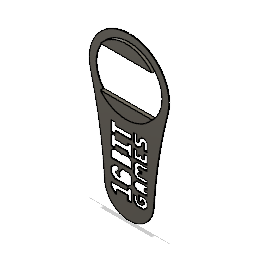
Poco X3 Phone Case Charm v1 (Autodesk Fusion 360 design; units mm, degrees)
Autodesk Fusion 360 part; units mm, degrees
note: some values were not read from the file. Chosen so that the rebuilt part matches the saved one: which pieces of a blend or face edit are solid. Set by a fixed rule: which sketch regions a step uses.
sketch "Sketch1" plane through (0, 0, 0) normal (0, 0, 1) x (1, 0, 0)
  circle A0 centre (0, 0) radius 18.4
  line L0 (-18.4, 0) -> (-13.8, 0)
  line L1 (-13.8, 0) -> (-13.8, -12.1705)
  line L2 (18.4, 0) -> (13.8, 0)
  line L3 (13.8, 0) -> (13.8, -12.1705)
  line L4 (0, -18.4) -> (0, -68.4)
  circle A1 centre (0, -54.6) radius 13.8
  line L5 (-13.8, -12.1705) -> (-13.8, -54.6)
  line L6 (13.8, -12.1705) -> (13.8, -54.6)
  circle A2 centre (0, 0) radius 22.4
  line L7 (-18.4, 0) -> (-22.4, 0)
  line L8 (18.4, 0) -> (22.4, 0)
  line L9 (0, 0) -> (0, 11.25)
  circle A3 centre (0, 0) radius 17.4
  line L10 (0, 11.25) -> (13.2739, 11.25)
  line L11 (13.2739, 11.25) -> (-13.2739, 11.25)
  line L12 (-13.2739, 11.25) -> (-13.2739, -11.25)
  line L13 (-13.2739, -11.25) -> (13.2739, -11.25)
  line L14 (13.2739, -11.25) -> (13.2739, 11.25)
  line L15 (-13.2739, 0) -> (-13.2739, -11.25)
  line L16 (-13.2739, -5.625) -> (-21.6822, -5.625)
  line L17 (-13.2739, -5.625) -> (21.6822, -5.625)
  arc A4 (-13.8, -54.6) -> (-21.6822, -5.625) centre (-276.7651, -71.8009) ccw
  arc A5 (21.6822, -5.625) -> (13.8, -54.6) centre (276.765, -71.8009) ccw
  dimension "d1" = 36.8
  dimension "d2" = 4.6
  dimension "d3" = 4.6
  dimension "d4" = 50
  dimension "d5" = 27.6
  dimension "d6" = 4
  dimension "d7" = 11.25
  dimension "d8" = -1
  dimension "d9" = 22.5
  constraint coincident A0.centre A2.centre
  constraint coincident A0 L0.start
  constraint horizontal L0
  constraint coincident A0 L1.end
  constraint perpendicular L0 L1
  constraint coincident A0 L2.start
  constraint perpendicular L1 L2
  constraint coincident A0 L3.end
  constraint perpendicular L2 L3
  constraint coincident A0 L4.start
  constraint vertical L4
  constraint coincident L4.end A1
  constraint coincident A1 L5.end
  constraint tangent A1 L5
  constraint parallel L1 L5
  constraint coincident A1 L6.end
  constraint tangent A1 L6
  constraint parallel L3 L6
  constraint coincident A2 L7.end
  constraint parallel L0 L7
  constraint coincident A2 L8.end
  constraint parallel L2 L8
  constraint vertical L9
  constraint coincident A3 L10.end
  constraint perpendicular L9 L10
  constraint horizontal L11
  constraint vertical L12
  constraint horizontal L13
  constraint vertical L14
  constraint coincident A3 L12.end
  constraint midpoint L12 L15.start
  constraint midpoint L15 L16.start
  constraint coincident A2 L16.end
  constraint perpendicular L15 L16
  constraint coincident A2 L17.end
  constraint parallel L16 L17
  constraint tangent A2 A4
  constraint tangent A2 A5
  measures "d1" diameter of A0
  measures "d2" distance of L0.start L0.end
  measures "d3" distance of L2.start L2.end
  measures "d4" distance of L4.start L4.end
  measures "d5" diameter of A1
  measures "d7" distance of A0.centre L9.end
  measures "d9" distance of L10.end L13.end
extrude "Extrude1" add sketch "Sketch1" along normal blind 0.8 contours A0 L0 L2 A3 | A0 A2 L8 L17 | A0 L2 A3 L17 | A0 A2 L7 L8 | A0 L0 A3 L16 | A0 A2 L7 L16 | A0 L6 A2 L17 | A0 L3 A3 L17 | A0 L1 A3 L16 | A0 L5 A2 L16 | A0 L4 L6 A2 | A0 L1 L3 A3 | L6 A2 A5 | A3 L10 L11 | A0 L4 L5 A2 | L5 A2 A4 | L4 A1 L6 A2 | L4 A1 | L4 A1 L5 A2 | L4 A1 | A3 L13 makes body 1
extrude "Extrude2" add sketch "Sketch1" along normal blind 2 contours A0 L0 L2 A3 | A0 L2 A3 L17 | A0 L0 A3 L16 | A0 L3 A3 L17 | A0 L1 A3 L16 | A0 L1 L3 A3 | A3 L10 L11 | A3 L13 bodies 1
extrude "Extrude3" cut 1 faces at (-0.4583, -31.5299, 0.8) along direction (0, 0, -1) blind 0.4 on bodies 1 bodies 1
sketch "Sketch2" plane through (0, 0, 0.4) normal (0, 0, 1) x (1, 0, 0)
  circle A0 centre (0, 0) radius 18.4
  arc A1 (-13.8, -54.6) -> (13.8, -54.6) centre (0, -54.6) ccw
  arc A2 (21.6822, -5.625) -> (13.8, -54.6) centre (276.765, -71.8009) ccw
  arc A3 (21.6822, -5.625) -> (-21.6822, -5.625) centre (0, 0) ccw
  arc A4 (-13.8, -54.6) -> (-21.6822, -5.625) centre (-276.7651, -71.8009) ccw
  line L0 (-10.0235, -64.9162) -> (-9.6068, -64.9162)
  line L1 (-9.6068, -64.9162) -> (-9.6068, -65.3329)
  line L2 (-9.6068, -65.3329) -> (-9.1902, -65.3329)
  line L3 (-9.1902, -65.3329) -> (-9.1902, -65.7495)
  line L4 (-9.1902, -65.7495) -> (-8.7735, -65.7495)
  line L5 (-8.7735, -65.7495) -> (-8.7735, -66.1662)
  line L6 (-8.7735, -66.1662) -> (-8.3568, -66.1662)
  line L7 (-8.3568, -66.1662) -> (-8.3568, -66.5829)
  line L8 (-8.3568, -66.5829) -> (-7.9402, -66.5829)
  line L9 (-7.9402, -66.5829) -> (-7.9402, -66.9995)
  line L10 (-7.9402, -66.9995) -> (-7.1068, -66.9995)
  line L11 (-7.1068, -66.9995) -> (-7.1068, -64.4995)
  line L12 (-7.1068, -64.4995) -> (-0.8568, -64.4995)
  line L13 (-0.8568, -64.4995) -> (-0.8568, -66.9995)
  line L14 (-0.8568, -66.9995) -> (1.2265, -66.9995)
  line L15 (1.2265, -66.9995) -> (1.2265, -60.7495)
  line L16 (1.2265, -60.7495) -> (-0.8568, -60.7495)
  line L17 (-0.8568, -60.7495) -> (-0.8568, -62.4162)
  line L18 (-0.8568, -62.4162) -> (-10.0235, -62.4162)
  line L19 (-10.0235, -62.4162) -> (-10.0235, -64.9162)
  line L20 (-10.0235, -58.2495) -> (-9.6068, -58.2495)
  line L21 (-9.6068, -58.2495) -> (-9.6068, -58.6662)
  line L22 (-9.6068, -58.6662) -> (-9.1902, -58.6662)
  line L23 (-9.1902, -58.6662) -> (-9.1902, -59.0829)
  line L24 (-9.1902, -59.0829) -> (-8.7735, -59.0829)
  line L25 (-8.7735, -59.0829) -> (-8.7735, -59.4995)
  line L26 (-8.7735, -59.4995) -> (-8.3568, -59.4995)
  line L27 (-8.3568, -59.4995) -> (-8.3568, -59.9162)
  line L28 (-8.3568, -59.9162) -> (-0.4402, -59.9162)
  line L29 (-0.4402, -59.9162) -> (-0.4402, -59.4995)
  line L30 (-0.4402, -59.4995) -> (-0.0235, -59.4995)
  line L31 (-0.0235, -59.4995) -> (-0.0235, -59.0829)
  line L32 (-0.0235, -59.0829) -> (0.3932, -59.0829)
  line L33 (0.3932, -59.0829) -> (0.3932, -58.6662)
  line L34 (0.3932, -58.6662) -> (0.8098, -58.6662)
  line L35 (0.8098, -58.6662) -> (0.8098, -58.2495)
  line L36 (0.8098, -58.2495) -> (1.2265, -58.2495)
  line L37 (1.2265, -58.2495) -> (1.2265, -54.4995)
  line L38 (1.2265, -54.4995) -> (0.8098, -54.4995)
  line L39 (0.8098, -54.4995) -> (0.8098, -54.0829)
  line L40 (0.8098, -54.0829) -> (0.3932, -54.0829)
  line L41 (0.3932, -54.0829) -> (0.3932, -53.6662)
  line L42 (0.3932, -53.6662) -> (-0.0235, -53.6662)
  line L43 (-0.0235, -53.6662) -> (-0.0235, -53.2495)
  line L44 (-0.0235, -53.2495) -> (-3.7735, -53.2495)
  line L45 (-3.7735, -53.2495) -> (-3.7735, -53.6662)
  line L46 (-3.7735, -53.6662) -> (-4.1902, -53.6662)
  line L47 (-4.1902, -53.6662) -> (-4.1902, -54.0829)
  line L48 (-4.1902, -54.0829) -> (-4.6068, -54.0829)
  line L49 (-4.6068, -54.0829) -> (-4.6068, -54.4995)
  line L50 (-4.6068, -54.4995) -> (-5.0235, -54.4995)
  line L51 (-5.0235, -54.4995) -> (-5.0235, -54.9162)
  line L52 (-5.0235, -54.9162) -> (-5.4402, -54.9162)
  line L53 (-5.4402, -54.9162) -> (-5.4402, -57.4162)
  line L54 (-5.4402, -57.4162) -> (-5.0235, -57.4162)
  line L55 (-5.0235, -57.4162) -> (-5.0235, -57.8329)
  line L56 (-5.0235, -57.8329) -> (-6.6902, -57.8329)
  line L57 (-6.6902, -57.8329) -> (-6.6902, -57.4162)
  line L58 (-6.6902, -57.4162) -> (-7.1068, -57.4162)
  line L59 (-7.1068, -57.4162) -> (-7.1068, -56.9995)
  line L60 (-7.1068, -56.9995) -> (-7.5235, -56.9995)
  line L61 (-7.5235, -56.9995) -> (-7.5235, -55.7495)
  line L62 (-7.5235, -55.7495) -> (-7.1068, -55.7495)
  line L63 (-7.1068, -55.7495) -> (-7.1068, -55.3329)
  line L64 (-7.1068, -55.3329) -> (-6.2735, -55.3329)
  line L65 (-6.2735, -55.3329) -> (-6.2735, -53.2495)
  line L66 (-6.2735, -53.2495) -> (-8.3568, -53.2495)
  line L67 (-8.3568, -53.2495) -> (-8.3568, -53.6662)
  line L68 (-8.3568, -53.6662) -> (-8.7735, -53.6662)
  line L69 (-8.7735, -53.6662) -> (-8.7735, -54.0829)
  line L70 (-8.7735, -54.0829) -> (-9.1902, -54.0829)
  line L71 (-9.1902, -54.0829) -> (-9.1902, -54.4995)
  line L72 (-9.1902, -54.4995) -> (-9.6068, -54.4995)
  line L73 (-9.6068, -54.4995) -> (-9.6068, -54.9162)
  line L74 (-9.6068, -54.9162) -> (-10.0235, -54.9162)
  line L75 (-10.0235, -54.9162) -> (-10.0235, -58.2495)
  line L76 (-10.0235, -50.7495) -> (1.2265, -50.7495)
  line L77 (1.2265, -50.7495) -> (1.2265, -46.9995)
  line L78 (1.2265, -46.9995) -> (0.8098, -46.9995)
  line L79 (0.8098, -46.9995) -> (0.8098, -46.5829)
  line L80 (0.8098, -46.5829) -> (0.3932, -46.5829)
  line L81 (0.3932, -46.5829) -> (0.3932, -46.1662)
  line L82 (0.3932, -46.1662) -> (-0.0235, -46.1662)
  line L83 (-0.0235, -46.1662) -> (-0.0235, -45.7495)
  line L84 (-0.0235, -45.7495) -> (-3.7735, -45.7495)
  line L85 (-3.7735, -45.7495) -> (-3.7735, -46.1662)
  line L86 (-3.7735, -46.1662) -> (-4.1902, -46.1662)
  line L87 (-4.1902, -46.1662) -> (-4.1902, -46.5829)
  line L88 (-4.1902, -46.5829) -> (-4.6068, -46.5829)
  line L89 (-4.6068, -46.5829) -> (-4.6068, -46.1662)
  line L90 (-4.6068, -46.1662) -> (-5.0235, -46.1662)
  line L91 (-5.0235, -46.1662) -> (-5.0235, -45.7495)
  line L92 (-5.0235, -45.7495) -> (-8.7735, -45.7495)
  line L93 (-8.7735, -45.7495) -> (-8.7735, -46.1662)
  line L94 (-8.7735, -46.1662) -> (-9.1902, -46.1662)
  line L95 (-9.1902, -46.1662) -> (-9.1902, -46.5829)
  line L96 (-9.1902, -46.5829) -> (-9.6068, -46.5829)
  line L97 (-9.6068, -46.5829) -> (-9.6068, -46.9995)
  line L98 (-9.6068, -46.9995) -> (-10.0235, -46.9995)
  line L99 (-10.0235, -46.9995) -> (-10.0235, -50.7495)
  line L100 (-10.0235, -44.9162) -> (-7.9402, -44.9162)
  line L101 (-7.9402, -44.9162) -> (-7.9402, -43.2495)
  line L102 (-7.9402, -43.2495) -> (-0.8568, -43.2495)
  line L103 (-0.8568, -43.2495) -> (-0.8568, -44.9162)
  line L104 (-0.8568, -44.9162) -> (1.2265, -44.9162)
  line L105 (1.2265, -44.9162) -> (1.2265, -39.0829)
  line L106 (1.2265, -39.0829) -> (-0.8568, -39.0829)
  line L107 (-0.8568, -39.0829) -> (-0.8568, -40.7495)
  line L108 (-0.8568, -40.7495) -> (-7.9402, -40.7495)
  line L109 (-7.9402, -40.7495) -> (-7.9402, -39.0829)
  line L110 (-7.9402, -39.0829) -> (-10.0235, -39.0829)
  line L111 (-10.0235, -39.0829) -> (-10.0235, -44.9162)
  line L112 (-10.0235, -38.2495) -> (-7.9402, -38.2495)
  line L113 (-7.9402, -38.2495) -> (-7.9402, -36.5829)
  line L114 (-7.9402, -36.5829) -> (1.2265, -36.5829)
  line L115 (1.2265, -36.5829) -> (1.2265, -34.0829)
  line L116 (1.2265, -34.0829) -> (-7.9402, -34.0829)
  line L117 (-7.9402, -34.0829) -> (-7.9402, -32.4162)
  line L118 (-7.9402, -32.4162) -> (-10.0235, -32.4162)
  line L119 (-10.0235, -32.4162) -> (-10.0235, -38.2495)
  line L120 (-9.6068, -62.8329) -> (-0.4402, -62.8329)
  line L121 (-0.4402, -62.8329) -> (-0.4402, -61.1662)
  line L122 (-0.4402, -61.1662) -> (0.8098, -61.1662)
  line L123 (0.8098, -61.1662) -> (0.8098, -66.5829)
  line L124 (0.8098, -66.5829) -> (-0.4402, -66.5829)
  line L125 (-0.4402, -66.5829) -> (-0.4402, -64.0829)
  line L126 (-0.4402, -64.0829) -> (-7.5235, -64.0829)
  line L127 (-7.5235, -64.0829) -> (-7.5235, -66.1662)
  line L128 (-7.5235, -66.1662) -> (-7.9402, -66.1662)
  line L129 (-7.9402, -66.1662) -> (-7.9402, -65.7495)
  line L130 (-7.9402, -65.7495) -> (-8.3568, -65.7495)
  line L131 (-8.3568, -65.7495) -> (-8.3568, -65.3329)
  line L132 (-8.3568, -65.3329) -> (-8.7735, -65.3329)
  line L133 (-8.7735, -65.3329) -> (-8.7735, -64.9162)
  line L134 (-8.7735, -64.9162) -> (-9.1902, -64.9162)
  line L135 (-9.1902, -64.9162) -> (-9.1902, -64.4995)
  line L136 (-9.1902, -64.4995) -> (-9.6068, -64.4995)
  line L137 (-9.6068, -64.4995) -> (-9.6068, -62.8329)
  line L138 (-9.6068, -55.3329) -> (-9.1902, -55.3329)
  line L139 (-9.1902, -55.3329) -> (-9.1902, -54.9162)
  line L140 (-9.1902, -54.9162) -> (-8.7735, -54.9162)
  line L141 (-8.7735, -54.9162) -> (-8.7735, -54.4995)
  line L142 (-8.7735, -54.4995) -> (-8.3568, -54.4995)
  line L143 (-8.3568, -54.4995) -> (-8.3568, -54.0829)
  line L144 (-8.3568, -54.0829) -> (-7.9402, -54.0829)
  line L145 (-7.9402, -54.0829) -> (-7.9402, -53.6662)
  line L146 (-7.9402, -53.6662) -> (-6.6902, -53.6662)
  line L147 (-6.6902, -53.6662) -> (-6.6902, -54.9162)
  line L148 (-6.6902, -54.9162) -> (-7.5235, -54.9162)
  line L149 (-7.5235, -54.9162) -> (-7.5235, -55.3329)
  line L150 (-7.5235, -55.3329) -> (-7.9402, -55.3329)
  line L151 (-7.9402, -55.3329) -> (-7.9402, -57.4162)
  line L152 (-7.9402, -57.4162) -> (-7.5235, -57.4162)
  line L153 (-7.5235, -57.4162) -> (-7.5235, -57.8329)
  line L154 (-7.5235, -57.8329) -> (-7.1068, -57.8329)
  line L155 (-7.1068, -57.8329) -> (-7.1068, -58.2495)
  line L156 (-7.1068, -58.2495) -> (-4.1902, -58.2495)
  line L157 (-4.1902, -58.2495) -> (-4.1902, -57.4162)
  line L158 (-4.1902, -57.4162) -> (-4.6068, -57.4162)
  line L159 (-4.6068, -57.4162) -> (-4.6068, -56.9995)
  line L160 (-4.6068, -56.9995) -> (-5.0235, -56.9995)
  line L161 (-5.0235, -56.9995) -> (-5.0235, -55.3329)
  line L162 (-5.0235, -55.3329) -> (-4.6068, -55.3329)
  line L163 (-4.6068, -55.3329) -> (-4.6068, -54.9162)
  line L164 (-4.6068, -54.9162) -> (-4.1902, -54.9162)
  line L165 (-4.1902, -54.9162) -> (-4.1902, -54.4995)
  line L166 (-4.1902, -54.4995) -> (-3.7735, -54.4995)
  line L167 (-3.7735, -54.4995) -> (-3.7735, -54.0829)
  line L168 (-3.7735, -54.0829) -> (-3.3568, -54.0829)
  line L169 (-3.3568, -54.0829) -> (-3.3568, -53.6662)
  line L170 (-3.3568, -53.6662) -> (-0.4402, -53.6662)
  line L171 (-0.4402, -53.6662) -> (-0.4402, -54.0829)
  line L172 (-0.4402, -54.0829) -> (-0.0235, -54.0829)
  line L173 (-0.0235, -54.0829) -> (-0.0235, -54.4995)
  line L174 (-0.0235, -54.4995) -> (0.3932, -54.4995)
  line L175 (0.3932, -54.4995) -> (0.3932, -54.9162)
  line L176 (0.3932, -54.9162) -> (0.8098, -54.9162)
  line L177 (0.8098, -54.9162) -> (0.8098, -57.8329)
  line L178 (0.8098, -57.8329) -> (0.3932, -57.8329)
  line L179 (0.3932, -57.8329) -> (0.3932, -58.2495)
  line L180 (0.3932, -58.2495) -> (-0.0235, -58.2495)
  line L181 (-0.0235, -58.2495) -> (-0.0235, -58.6662)
  line L182 (-0.0235, -58.6662) -> (-0.4402, -58.6662)
  line L183 (-0.4402, -58.6662) -> (-0.4402, -59.0829)
  line L184 (-0.4402, -59.0829) -> (-0.8568, -59.0829)
  line L185 (-0.8568, -59.0829) -> (-0.8568, -59.4995)
  line L186 (-0.8568, -59.4995) -> (-7.9402, -59.4995)
  line L187 (-7.9402, -59.4995) -> (-7.9402, -59.0829)
  line L188 (-7.9402, -59.0829) -> (-8.3568, -59.0829)
  line L189 (-8.3568, -59.0829) -> (-8.3568, -58.6662)
  line L190 (-8.3568, -58.6662) -> (-8.7735, -58.6662)
  line L191 (-8.7735, -58.6662) -> (-8.7735, -58.2495)
  line L192 (-8.7735, -58.2495) -> (-9.1902, -58.2495)
  line L193 (-9.1902, -58.2495) -> (-9.1902, -57.8329)
  line L194 (-9.1902, -57.8329) -> (-9.6068, -57.8329)
  line L195 (-9.6068, -57.8329) -> (-9.6068, -55.3329)
  line L196 (-9.6068, -47.4162) -> (-9.1902, -47.4162)
  line L197 (-9.1902, -47.4162) -> (-9.1902, -46.9995)
  line L198 (-9.1902, -46.9995) -> (-8.7735, -46.9995)
  line L199 (-8.7735, -46.9995) -> (-8.7735, -46.5829)
  line L200 (-8.7735, -46.5829) -> (-8.3568, -46.5829)
  line L201 (-8.3568, -46.5829) -> (-8.3568, -46.1662)
  line L202 (-8.3568, -46.1662) -> (-5.4402, -46.1662)
  line L203 (-5.4402, -46.1662) -> (-5.4402, -46.5829)
  line L204 (-5.4402, -46.5829) -> (-5.0235, -46.5829)
  line L205 (-5.0235, -46.5829) -> (-5.0235, -47.8329)
  line L206 (-5.0235, -47.8329) -> (-4.6068, -47.8329)
  line L207 (-4.6068, -47.8329) -> (-4.6068, -47.4162)
  line L208 (-4.6068, -47.4162) -> (-4.1902, -47.4162)
  line L209 (-4.1902, -47.4162) -> (-4.1902, -46.9995)
  line L210 (-4.1902, -46.9995) -> (-3.7735, -46.9995)
  line L211 (-3.7735, -46.9995) -> (-3.7735, -46.5829)
  line L212 (-3.7735, -46.5829) -> (-3.3568, -46.5829)
  line L213 (-3.3568, -46.5829) -> (-3.3568, -46.1662)
  line L214 (-3.3568, -46.1662) -> (-0.4402, -46.1662)
  line L215 (-0.4402, -46.1662) -> (-0.4402, -46.5829)
  line L216 (-0.4402, -46.5829) -> (-0.0235, -46.5829)
  line L217 (-0.0235, -46.5829) -> (-0.0235, -46.9995)
  line L218 (-0.0235, -46.9995) -> (0.3932, -46.9995)
  line L219 (0.3932, -46.9995) -> (0.3932, -47.4162)
  line L220 (0.3932, -47.4162) -> (0.8098, -47.4162)
  line L221 (0.8098, -47.4162) -> (0.8098, -50.3329)
  line L222 (0.8098, -50.3329) -> (-9.6068, -50.3329)
  line L223 (-9.6068, -50.3329) -> (-9.6068, -47.4162)
  line L224 (-9.6068, -39.4995) -> (-8.3568, -39.4995)
  line L225 (-8.3568, -39.4995) -> (-8.3568, -41.1662)
  line L226 (-8.3568, -41.1662) -> (-0.4402, -41.1662)
  line L227 (-0.4402, -41.1662) -> (-0.4402, -39.4995)
  line L228 (-0.4402, -39.4995) -> (0.8098, -39.4995)
  line L229 (0.8098, -39.4995) -> (0.8098, -44.4995)
  line L230 (0.8098, -44.4995) -> (-0.4402, -44.4995)
  line L231 (-0.4402, -44.4995) -> (-0.4402, -42.8329)
  line L232 (-0.4402, -42.8329) -> (-8.3568, -42.8329)
  line L233 (-8.3568, -42.8329) -> (-8.3568, -44.4995)
  line L234 (-8.3568, -44.4995) -> (-9.6068, -44.4995)
  line L235 (-9.6068, -44.4995) -> (-9.6068, -39.4995)
  line L236 (-9.6068, -32.8329) -> (-8.3568, -32.8329)
  line L237 (-8.3568, -32.8329) -> (-8.3568, -34.4995)
  line L238 (-8.3568, -34.4995) -> (0.8098, -34.4995)
  line L239 (0.8098, -34.4995) -> (0.8098, -36.1662)
  line L240 (0.8098, -36.1662) -> (-8.3568, -36.1662)
  line L241 (-8.3568, -36.1662) -> (-8.3568, -37.8329)
  line L242 (-8.3568, -37.8329) -> (-9.6068, -37.8329)
  line L243 (-9.6068, -37.8329) -> (-9.6068, -32.8329)
  line L244 (-8.7735, -49.4995) -> (-5.8568, -49.4995)
  line L245 (-5.8568, -49.4995) -> (-5.8568, -47.8329)
  line L246 (-5.8568, -47.8329) -> (-6.2735, -47.8329)
  line L247 (-6.2735, -47.8329) -> (-6.2735, -47.4162)
  line L248 (-6.2735, -47.4162) -> (-8.3568, -47.4162)
  line L249 (-8.3568, -47.4162) -> (-8.3568, -47.8329)
  line L250 (-8.3568, -47.8329) -> (-8.7735, -47.8329)
  line L251 (-8.7735, -47.8329) -> (-8.7735, -49.4995)
  line L252 (-8.3568, -48.2495) -> (-7.9402, -48.2495)
  line L253 (-7.9402, -48.2495) -> (-7.9402, -47.8329)
  line L254 (-7.9402, -47.8329) -> (-6.6902, -47.8329)
  line L255 (-6.6902, -47.8329) -> (-6.6902, -48.2495)
  line L256 (-6.6902, -48.2495) -> (-6.2735, -48.2495)
  line L257 (-6.2735, -48.2495) -> (-6.2735, -49.0829)
  line L258 (-6.2735, -49.0829) -> (-8.3568, -49.0829)
  line L259 (-8.3568, -49.0829) -> (-8.3568, -48.2495)
  line L260 (-3.7735, -57.4162) -> (-3.3568, -57.4162)
  line L261 (-3.3568, -57.4162) -> (-3.3568, -57.8329)
  line L262 (-3.3568, -57.8329) -> (-2.9402, -57.8329)
  line L263 (-2.9402, -57.8329) -> (-2.9402, -58.2495)
  line L264 (-2.9402, -58.2495) -> (-0.8568, -58.2495)
  line L265 (-0.8568, -58.2495) -> (-0.8568, -57.8329)
  line L266 (-0.8568, -57.8329) -> (-0.4402, -57.8329)
  line L267 (-0.4402, -57.8329) -> (-0.4402, -57.4162)
  line L268 (-0.4402, -57.4162) -> (-0.0235, -57.4162)
  line L269 (-0.0235, -57.4162) -> (-0.0235, -55.7495)
  line L270 (-0.0235, -55.7495) -> (-0.4402, -55.7495)
  line L271 (-0.4402, -55.7495) -> (-0.4402, -55.3329)
  line L272 (-0.4402, -55.3329) -> (-0.8568, -55.3329)
  line L273 (-0.8568, -55.3329) -> (-0.8568, -54.9162)
  line L274 (-0.8568, -54.9162) -> (-2.9402, -54.9162)
  line L275 (-2.9402, -54.9162) -> (-2.9402, -55.3329)
  line L276 (-2.9402, -55.3329) -> (-3.3568, -55.3329)
  line L277 (-3.3568, -55.3329) -> (-3.3568, -55.7495)
  line L278 (-3.3568, -55.7495) -> (-3.7735, -55.7495)
  line L279 (-3.7735, -55.7495) -> (-3.7735, -57.4162)
  line L280 (-3.7735, -49.4995) -> (-0.4402, -49.4995)
  line L281 (-0.4402, -49.4995) -> (-0.4402, -47.8329)
  line L282 (-0.4402, -47.8329) -> (-0.8568, -47.8329)
  line L283 (-0.8568, -47.8329) -> (-0.8568, -47.4162)
  line L284 (-0.8568, -47.4162) -> (-3.3568, -47.4162)
  line L285 (-3.3568, -47.4162) -> (-3.3568, -47.8329)
  line L286 (-3.3568, -47.8329) -> (-3.7735, -47.8329)
  line L287 (-3.7735, -47.8329) -> (-3.7735, -49.4995)
  line L288 (-3.3568, -56.1662) -> (-2.9402, -56.1662)
  line L289 (-2.9402, -56.1662) -> (-2.9402, -55.7495)
  line L290 (-2.9402, -55.7495) -> (-2.5235, -55.7495)
  line L291 (-2.5235, -55.7495) -> (-2.5235, -55.3329)
  line L292 (-2.5235, -55.3329) -> (-1.2735, -55.3329)
  line L293 (-1.2735, -55.3329) -> (-1.2735, -55.7495)
  line L294 (-1.2735, -55.7495) -> (-0.8568, -55.7495)
  line L295 (-0.8568, -55.7495) -> (-0.8568, -56.1662)
  line L296 (-0.8568, -56.1662) -> (-0.4402, -56.1662)
  line L297 (-0.4402, -56.1662) -> (-0.4402, -56.9995)
  line L298 (-0.4402, -56.9995) -> (-0.8568, -56.9995)
  line L299 (-0.8568, -56.9995) -> (-0.8568, -57.4162)
  line L300 (-0.8568, -57.4162) -> (-1.2735, -57.4162)
  line L301 (-1.2735, -57.4162) -> (-1.2735, -57.8329)
  line L302 (-1.2735, -57.8329) -> (-2.5235, -57.8329)
  line L303 (-2.5235, -57.8329) -> (-2.5235, -57.4162)
  line L304 (-2.5235, -57.4162) -> (-2.9402, -57.4162)
  line L305 (-2.9402, -57.4162) -> (-2.9402, -56.9995)
  line L306 (-2.9402, -56.9995) -> (-3.3568, -56.9995)
  line L307 (-3.3568, -56.9995) -> (-3.3568, -56.1662)
  line L308 (-3.3568, -48.2495) -> (-2.9402, -48.2495)
  line L309 (-2.9402, -48.2495) -> (-2.9402, -47.8329)
  line L310 (-2.9402, -47.8329) -> (-1.2735, -47.8329)
  line L311 (-1.2735, -47.8329) -> (-1.2735, -48.2495)
  line L312 (-1.2735, -48.2495) -> (-0.8568, -48.2495)
  line L313 (-0.8568, -48.2495) -> (-0.8568, -49.0829)
  line L314 (-0.8568, -49.0829) -> (-3.3568, -49.0829)
  line L315 (-3.3568, -49.0829) -> (-3.3568, -48.2495)
  line L316 (2.4765, -65.3329) -> (2.8932, -65.3329)
  line L317 (2.8932, -65.3329) -> (2.8932, -65.7495)
  line L318 (2.8932, -65.7495) -> (3.3098, -65.7495)
  line L319 (3.3098, -65.7495) -> (3.3098, -66.1662)
  line L320 (3.3098, -66.1662) -> (3.7265, -66.1662)
  line L321 (3.7265, -66.1662) -> (3.7265, -66.5829)
  line L322 (3.7265, -66.5829) -> (4.1432, -66.5829)
  line L323 (4.1432, -66.5829) -> (4.1432, -66.9995)
  line L324 (4.1432, -66.9995) -> (8.3098, -66.9995)
  line L325 (8.3098, -66.9995) -> (8.3098, -66.5829)
  line L326 (8.3098, -66.5829) -> (8.7265, -66.5829)
  line L327 (8.7265, -66.5829) -> (8.7265, -66.1662)
  line L328 (8.7265, -66.1662) -> (9.1432, -66.1662)
  line L329 (9.1432, -66.1662) -> (9.1432, -65.7495)
  line L330 (9.1432, -65.7495) -> (9.5598, -65.7495)
  line L331 (9.5598, -65.7495) -> (9.5598, -65.3329)
  line L332 (9.5598, -65.3329) -> (9.9765, -65.3329)
  line L333 (9.9765, -65.3329) -> (9.9765, -62.4162)
  line L334 (9.9765, -62.4162) -> (9.5598, -62.4162)
  line L335 (9.5598, -62.4162) -> (9.5598, -61.9995)
  line L336 (9.5598, -61.9995) -> (9.1432, -61.9995)
  line L337 (9.1432, -61.9995) -> (9.1432, -61.5829)
  line L338 (9.1432, -61.5829) -> (8.7265, -61.5829)
  line L339 (8.7265, -61.5829) -> (8.7265, -61.1662)
  line L340 (8.7265, -61.1662) -> (5.3932, -61.1662)
  line L341 (5.3932, -61.1662) -> (5.3932, -64.0829)
  line L342 (5.3932, -64.0829) -> (7.0598, -64.0829)
  line L343 (7.0598, -64.0829) -> (7.0598, -62.4162)
  line L344 (7.0598, -62.4162) -> (7.4765, -62.4162)
  line L345 (7.4765, -62.4162) -> (7.4765, -62.8329)
  line L346 (7.4765, -62.8329) -> (7.8932, -62.8329)
  line L347 (7.8932, -62.8329) -> (7.8932, -63.2495)
  line L348 (7.8932, -63.2495) -> (8.3098, -63.2495)
  line L349 (8.3098, -63.2495) -> (8.3098, -64.4995)
  line L350 (8.3098, -64.4995) -> (7.8932, -64.4995)
  line L351 (7.8932, -64.4995) -> (7.8932, -64.9162)
  line L352 (7.8932, -64.9162) -> (7.4765, -64.9162)
  line L353 (7.4765, -64.9162) -> (7.4765, -65.3329)
  line L354 (7.4765, -65.3329) -> (4.9765, -65.3329)
  line L355 (4.9765, -65.3329) -> (4.9765, -64.9162)
  line L356 (4.9765, -64.9162) -> (4.5598, -64.9162)
  line L357 (4.5598, -64.9162) -> (4.5598, -64.4995)
  line L358 (4.5598, -64.4995) -> (4.1432, -64.4995)
  line L359 (4.1432, -64.4995) -> (4.1432, -62.4162)
  line L360 (4.1432, -62.4162) -> (2.4765, -62.4162)
  line L361 (2.4765, -62.4162) -> (2.4765, -65.3329)
  line L362 (2.4765, -57.8329) -> (2.8932, -57.8329)
  line L363 (2.8932, -57.8329) -> (2.8932, -58.2495)
  line L364 (2.8932, -58.2495) -> (3.3098, -58.2495)
  line L365 (3.3098, -58.2495) -> (3.3098, -58.6662)
  line L366 (3.3098, -58.6662) -> (3.7265, -58.6662)
  line L367 (3.7265, -58.6662) -> (3.7265, -59.0829)
  line L368 (3.7265, -59.0829) -> (4.1432, -59.0829)
  line L369 (4.1432, -59.0829) -> (4.1432, -59.4995)
  line L370 (4.1432, -59.4995) -> (9.9765, -59.4995)
  line L371 (9.9765, -59.4995) -> (9.9765, -57.8329)
  line L372 (9.9765, -57.8329) -> (8.3098, -57.8329)
  line L373 (8.3098, -57.8329) -> (8.3098, -56.5829)
  line L374 (8.3098, -56.5829) -> (9.9765, -56.5829)
  line L375 (9.9765, -56.5829) -> (9.9765, -54.9162)
  line L376 (9.9765, -54.9162) -> (4.1432, -54.9162)
  line L377 (4.1432, -54.9162) -> (4.1432, -55.3329)
  line L378 (4.1432, -55.3329) -> (3.7265, -55.3329)
  line L379 (3.7265, -55.3329) -> (3.7265, -55.7495)
  line L380 (3.7265, -55.7495) -> (3.3098, -55.7495)
  line L381 (3.3098, -55.7495) -> (3.3098, -56.1662)
  line L382 (3.3098, -56.1662) -> (2.8932, -56.1662)
  line L383 (2.8932, -56.1662) -> (2.8932, -56.5829)
  line L384 (2.8932, -56.5829) -> (2.4765, -56.5829)
  line L385 (2.4765, -56.5829) -> (2.4765, -57.8329)
  line L386 (2.4765, -51.9995) -> (2.8932, -51.9995)
  line L387 (2.8932, -51.9995) -> (2.8932, -52.4162)
  line L388 (2.8932, -52.4162) -> (3.3098, -52.4162)
  line L389 (3.3098, -52.4162) -> (3.3098, -52.8329)
  line L390 (3.3098, -52.8329) -> (3.7265, -52.8329)
  line L391 (3.7265, -52.8329) -> (3.7265, -53.2495)
  line L392 (3.7265, -53.2495) -> (4.1432, -53.2495)
  line L393 (4.1432, -53.2495) -> (4.1432, -53.6662)
  line L394 (4.1432, -53.6662) -> (9.9765, -53.6662)
  line L395 (9.9765, -53.6662) -> (9.9765, -51.9995)
  line L396 (9.9765, -51.9995) -> (4.9765, -51.9995)
  line L397 (4.9765, -51.9995) -> (4.9765, -51.5829)
  line L398 (4.9765, -51.5829) -> (4.5598, -51.5829)
  line L399 (4.5598, -51.5829) -> (4.5598, -50.7495)
  line L400 (4.5598, -50.7495) -> (4.9765, -50.7495)
  line L401 (4.9765, -50.7495) -> (4.9765, -50.3329)
  line L402 (4.9765, -50.3329) -> (7.0598, -50.3329)
  line L403 (7.0598, -50.3329) -> (7.0598, -49.0829)
  line L404 (7.0598, -49.0829) -> (4.9765, -49.0829)
  line L405 (4.9765, -49.0829) -> (4.9765, -48.6662)
  line L406 (4.9765, -48.6662) -> (4.5598, -48.6662)
  line L407 (4.5598, -48.6662) -> (4.5598, -47.8329)
  line L408 (4.5598, -47.8329) -> (4.9765, -47.8329)
  line L409 (4.9765, -47.8329) -> (4.9765, -47.4162)
  line L410 (4.9765, -47.4162) -> (9.9765, -47.4162)
  line L411 (9.9765, -47.4162) -> (9.9765, -45.7495)
  line L412 (9.9765, -45.7495) -> (4.1432, -45.7495)
  line L413 (4.1432, -45.7495) -> (4.1432, -46.1662)
  line L414 (4.1432, -46.1662) -> (3.7265, -46.1662)
  line L415 (3.7265, -46.1662) -> (3.7265, -46.5829)
  line L416 (3.7265, -46.5829) -> (3.3098, -46.5829)
  line L417 (3.3098, -46.5829) -> (3.3098, -46.9995)
  line L418 (3.3098, -46.9995) -> (2.8932, -46.9995)
  line L419 (2.8932, -46.9995) -> (2.8932, -47.4162)
  line L420 (2.8932, -47.4162) -> (2.4765, -47.4162)
  line L421 (2.4765, -47.4162) -> (2.4765, -49.0829)
  line L422 (2.4765, -49.0829) -> (2.8932, -49.0829)
  line L423 (2.8932, -49.0829) -> (2.8932, -49.4995)
  line L424 (2.8932, -49.4995) -> (3.3098, -49.4995)
  line L425 (3.3098, -49.4995) -> (3.3098, -49.9162)
  line L426 (3.3098, -49.9162) -> (2.8932, -49.9162)
  line L427 (2.8932, -49.9162) -> (2.8932, -50.3329)
  line L428 (2.8932, -50.3329) -> (2.4765, -50.3329)
  line L429 (2.4765, -50.3329) -> (2.4765, -51.9995)
  line L430 (2.4765, -44.4995) -> (9.9765, -44.4995)
  line L431 (9.9765, -44.4995) -> (9.9765, -39.9162)
  line L432 (9.9765, -39.9162) -> (8.3098, -39.9162)
  line L433 (8.3098, -39.9162) -> (8.3098, -42.8329)
  line L434 (8.3098, -42.8329) -> (7.0598, -42.8329)
  line L435 (7.0598, -42.8329) -> (7.0598, -41.5829)
  line L436 (7.0598, -41.5829) -> (5.3932, -41.5829)
  line L437 (5.3932, -41.5829) -> (5.3932, -42.8329)
  line L438 (5.3932, -42.8329) -> (4.1432, -42.8329)
  line L439 (4.1432, -42.8329) -> (4.1432, -39.9162)
  line L440 (4.1432, -39.9162) -> (2.4765, -39.9162)
  line L441 (2.4765, -39.9162) -> (2.4765, -44.4995)
  line L442 (2.4765, -36.9995) -> (2.8932, -36.9995)
  line L443 (2.8932, -36.9995) -> (2.8932, -37.4162)
  line L444 (2.8932, -37.4162) -> (3.3098, -37.4162)
  line L445 (3.3098, -37.4162) -> (3.3098, -37.8329)
  line L446 (3.3098, -37.8329) -> (3.7265, -37.8329)
  line L447 (3.7265, -37.8329) -> (3.7265, -38.2495)
  line L448 (3.7265, -38.2495) -> (5.3932, -38.2495)
  line L449 (5.3932, -38.2495) -> (5.3932, -37.8329)
  line L450 (5.3932, -37.8329) -> (5.8098, -37.8329)
  line L451 (5.8098, -37.8329) -> (5.8098, -37.4162)
  line L452 (5.8098, -37.4162) -> (6.2265, -37.4162)
  line L453 (6.2265, -37.4162) -> (6.2265, -36.9995)
  line L454 (6.2265, -36.9995) -> (6.6432, -36.9995)
  line L455 (6.6432, -36.9995) -> (6.6432, -36.5829)
  line L456 (6.6432, -36.5829) -> (7.0598, -36.5829)
  line L457 (7.0598, -36.5829) -> (7.0598, -34.9162)
  line L458 (7.0598, -34.9162) -> (7.4765, -34.9162)
  line L459 (7.4765, -34.9162) -> (7.4765, -34.4995)
  line L460 (7.4765, -34.4995) -> (8.3098, -34.4995)
  line L461 (8.3098, -34.4995) -> (8.3098, -38.2495)
  line L462 (8.3098, -38.2495) -> (9.9765, -38.2495)
  line L463 (9.9765, -38.2495) -> (9.9765, -33.6662)
  line L464 (9.9765, -33.6662) -> (9.5598, -33.6662)
  line L465 (9.5598, -33.6662) -> (9.5598, -33.2495)
  line L466 (9.5598, -33.2495) -> (9.1432, -33.2495)
  line L467 (9.1432, -33.2495) -> (9.1432, -32.8329)
  line L468 (9.1432, -32.8329) -> (8.7265, -32.8329)
  line L469 (8.7265, -32.8329) -> (8.7265, -32.4162)
  line L470 (8.7265, -32.4162) -> (7.0598, -32.4162)
  line L471 (7.0598, -32.4162) -> (7.0598, -32.8329)
  line L472 (7.0598, -32.8329) -> (6.6432, -32.8329)
  line L473 (6.6432, -32.8329) -> (6.6432, -33.2495)
  line L474 (6.6432, -33.2495) -> (6.2265, -33.2495)
  line L475 (6.2265, -33.2495) -> (6.2265, -33.6662)
  line L476 (6.2265, -33.6662) -> (5.8098, -33.6662)
  line L477 (5.8098, -33.6662) -> (5.8098, -34.0829)
  line L478 (5.8098, -34.0829) -> (5.3932, -34.0829)
  line L479 (5.3932, -34.0829) -> (5.3932, -35.7495)
  line L480 (5.3932, -35.7495) -> (4.9765, -35.7495)
  line L481 (4.9765, -35.7495) -> (4.9765, -36.1662)
  line L482 (4.9765, -36.1662) -> (4.1432, -36.1662)
  line L483 (4.1432, -36.1662) -> (4.1432, -32.4162)
  line L484 (4.1432, -32.4162) -> (2.4765, -32.4162)
  line L485 (2.4765, -32.4162) -> (2.4765, -36.9995)
  line L486 (2.8932, -62.8329) -> (3.7265, -62.8329)
  line L487 (3.7265, -62.8329) -> (3.7265, -64.9162)
  line L488 (3.7265, -64.9162) -> (4.1432, -64.9162)
  line L489 (4.1432, -64.9162) -> (4.1432, -65.3329)
  line L490 (4.1432, -65.3329) -> (4.5598, -65.3329)
  line L491 (4.5598, -65.3329) -> (4.5598, -65.7495)
  line L492 (4.5598, -65.7495) -> (7.8932, -65.7495)
  line L493 (7.8932, -65.7495) -> (7.8932, -65.3329)
  line L494 (7.8932, -65.3329) -> (8.3098, -65.3329)
  line L495 (8.3098, -65.3329) -> (8.3098, -64.9162)
  line L496 (8.3098, -64.9162) -> (8.7265, -64.9162)
  line L497 (8.7265, -64.9162) -> (8.7265, -62.8329)
  line L498 (8.7265, -62.8329) -> (8.3098, -62.8329)
  line L499 (8.3098, -62.8329) -> (8.3098, -62.4162)
  line L500 (8.3098, -62.4162) -> (7.8932, -62.4162)
  line L501 (7.8932, -62.4162) -> (7.8932, -61.9995)
  line L502 (7.8932, -61.9995) -> (6.6432, -61.9995)
  line L503 (6.6432, -61.9995) -> (6.6432, -63.6662)
  line L504 (6.6432, -63.6662) -> (5.8098, -63.6662)
  line L505 (5.8098, -63.6662) -> (5.8098, -61.5829)
  line L506 (5.8098, -61.5829) -> (8.3098, -61.5829)
  line L507 (8.3098, -61.5829) -> (8.3098, -61.9995)
  line L508 (8.3098, -61.9995) -> (8.7265, -61.9995)
  line L509 (8.7265, -61.9995) -> (8.7265, -62.4162)
  line L510 (8.7265, -62.4162) -> (9.1432, -62.4162)
  line L511 (9.1432, -62.4162) -> (9.1432, -62.8329)
  line L512 (9.1432, -62.8329) -> (9.5598, -62.8329)
  line L513 (9.5598, -62.8329) -> (9.5598, -64.9162)
  line L514 (9.5598, -64.9162) -> (9.1432, -64.9162)
  line L515 (9.1432, -64.9162) -> (9.1432, -65.3329)
  line L516 (9.1432, -65.3329) -> (8.7265, -65.3329)
  line L517 (8.7265, -65.3329) -> (8.7265, -65.7495)
  line L518 (8.7265, -65.7495) -> (8.3098, -65.7495)
  line L519 (8.3098, -65.7495) -> (8.3098, -66.1662)
  line L520 (8.3098, -66.1662) -> (7.8932, -66.1662)
  line L521 (7.8932, -66.1662) -> (7.8932, -66.5829)
  line L522 (7.8932, -66.5829) -> (4.5598, -66.5829)
  line L523 (4.5598, -66.5829) -> (4.5598, -66.1662)
  line L524 (4.5598, -66.1662) -> (4.1432, -66.1662)
  line L525 (4.1432, -66.1662) -> (4.1432, -65.7495)
  line L526 (4.1432, -65.7495) -> (3.7265, -65.7495)
  line L527 (3.7265, -65.7495) -> (3.7265, -65.3329)
  line L528 (3.7265, -65.3329) -> (3.3098, -65.3329)
  line L529 (3.3098, -65.3329) -> (3.3098, -64.9162)
  line L530 (3.3098, -64.9162) -> (2.8932, -64.9162)
  line L531 (2.8932, -64.9162) -> (2.8932, -62.8329)
  line L532 (2.8932, -56.9995) -> (3.3098, -56.9995)
  line L533 (3.3098, -56.9995) -> (3.3098, -56.5829)
  line L534 (3.3098, -56.5829) -> (3.7265, -56.5829)
  line L535 (3.7265, -56.5829) -> (3.7265, -56.1662)
  line L536 (3.7265, -56.1662) -> (4.1432, -56.1662)
  line L537 (4.1432, -56.1662) -> (4.1432, -55.7495)
  line L538 (4.1432, -55.7495) -> (4.5598, -55.7495)
  line L539 (4.5598, -55.7495) -> (4.5598, -55.3329)
  line L540 (4.5598, -55.3329) -> (9.5598, -55.3329)
  line L541 (9.5598, -55.3329) -> (9.5598, -56.1662)
  line L542 (9.5598, -56.1662) -> (7.8932, -56.1662)
  line L543 (7.8932, -56.1662) -> (7.8932, -58.2495)
  line L544 (7.8932, -58.2495) -> (9.5598, -58.2495)
  line L545 (9.5598, -58.2495) -> (9.5598, -59.0829)
  line L546 (9.5598, -59.0829) -> (4.5598, -59.0829)
  line L547 (4.5598, -59.0829) -> (4.5598, -58.6662)
  line L548 (4.5598, -58.6662) -> (4.1432, -58.6662)
  line L549 (4.1432, -58.6662) -> (4.1432, -58.2495)
  line L550 (4.1432, -58.2495) -> (3.7265, -58.2495)
  line L551 (3.7265, -58.2495) -> (3.7265, -57.8329)
  line L552 (3.7265, -57.8329) -> (3.3098, -57.8329)
  line L553 (3.3098, -57.8329) -> (3.3098, -57.4162)
  line L554 (3.3098, -57.4162) -> (2.8932, -57.4162)
  line L555 (2.8932, -57.4162) -> (2.8932, -56.9995)
  line L556 (2.8932, -50.7495) -> (3.3098, -50.7495)
  line L557 (3.3098, -50.7495) -> (3.3098, -50.3329)
  line L558 (3.3098, -50.3329) -> (3.7265, -50.3329)
  line L559 (3.7265, -50.3329) -> (3.7265, -49.9162)
  line L560 (3.7265, -49.9162) -> (4.1432, -49.9162)
  line L561 (4.1432, -49.9162) -> (4.1432, -49.4995)
  line L562 (4.1432, -49.4995) -> (3.7265, -49.4995)
  line L563 (3.7265, -49.4995) -> (3.7265, -49.0829)
  line L564 (3.7265, -49.0829) -> (3.3098, -49.0829)
  line L565 (3.3098, -49.0829) -> (3.3098, -48.6662)
  line L566 (3.3098, -48.6662) -> (2.8932, -48.6662)
  line L567 (2.8932, -48.6662) -> (2.8932, -47.8329)
  line L568 (2.8932, -47.8329) -> (3.3098, -47.8329)
  line L569 (3.3098, -47.8329) -> (3.3098, -47.4162)
  line L570 (3.3098, -47.4162) -> (3.7265, -47.4162)
  line L571 (3.7265, -47.4162) -> (3.7265, -46.9995)
  line L572 (3.7265, -46.9995) -> (4.1432, -46.9995)
  line L573 (4.1432, -46.9995) -> (4.1432, -46.5829)
  line L574 (4.1432, -46.5829) -> (4.5598, -46.5829)
  line L575 (4.5598, -46.5829) -> (4.5598, -46.1662)
  line L576 (4.5598, -46.1662) -> (9.5598, -46.1662)
  line L577 (9.5598, -46.1662) -> (9.5598, -46.9995)
  line L578 (9.5598, -46.9995) -> (4.5598, -46.9995)
  line L579 (4.5598, -46.9995) -> (4.5598, -47.4162)
  line L580 (4.5598, -47.4162) -> (4.1432, -47.4162)
  line L581 (4.1432, -47.4162) -> (4.1432, -47.8329)
  line L582 (4.1432, -47.8329) -> (3.7265, -47.8329)
  line L583 (3.7265, -47.8329) -> (3.7265, -48.6662)
  line L584 (3.7265, -48.6662) -> (4.1432, -48.6662)
  line L585 (4.1432, -48.6662) -> (4.1432, -49.0829)
  line L586 (4.1432, -49.0829) -> (4.5598, -49.0829)
  line L587 (4.5598, -49.0829) -> (4.5598, -49.4995)
  line L588 (4.5598, -49.4995) -> (6.6432, -49.4995)
  line L589 (6.6432, -49.4995) -> (6.6432, -49.9162)
  line L590 (6.6432, -49.9162) -> (4.5598, -49.9162)
  line L591 (4.5598, -49.9162) -> (4.5598, -50.3329)
  line L592 (4.5598, -50.3329) -> (4.1432, -50.3329)
  line L593 (4.1432, -50.3329) -> (4.1432, -50.7495)
  line L594 (4.1432, -50.7495) -> (3.7265, -50.7495)
  line L595 (3.7265, -50.7495) -> (3.7265, -51.5829)
  line L596 (3.7265, -51.5829) -> (4.1432, -51.5829)
  line L597 (4.1432, -51.5829) -> (4.1432, -51.9995)
  line L598 (4.1432, -51.9995) -> (4.5598, -51.9995)
  line L599 (4.5598, -51.9995) -> (4.5598, -52.4162)
  line L600 (4.5598, -52.4162) -> (9.5598, -52.4162)
  line L601 (9.5598, -52.4162) -> (9.5598, -53.2495)
  line L602 (9.5598, -53.2495) -> (4.5598, -53.2495)
  line L603 (4.5598, -53.2495) -> (4.5598, -52.8329)
  line L604 (4.5598, -52.8329) -> (4.1432, -52.8329)
  line L605 (4.1432, -52.8329) -> (4.1432, -52.4162)
  line L606 (4.1432, -52.4162) -> (3.7265, -52.4162)
  line L607 (3.7265, -52.4162) -> (3.7265, -51.9995)
  line L608 (3.7265, -51.9995) -> (3.3098, -51.9995)
  line L609 (3.3098, -51.9995) -> (3.3098, -51.5829)
  line L610 (3.3098, -51.5829) -> (2.8932, -51.5829)
  line L611 (2.8932, -51.5829) -> (2.8932, -50.7495)
  line L612 (2.8932, -40.3329) -> (3.7265, -40.3329)
  line L613 (3.7265, -40.3329) -> (3.7265, -43.2495)
  line L614 (3.7265, -43.2495) -> (5.8098, -43.2495)
  line L615 (5.8098, -43.2495) -> (5.8098, -41.9995)
  line L616 (5.8098, -41.9995) -> (6.6432, -41.9995)
  line L617 (6.6432, -41.9995) -> (6.6432, -43.2495)
  line L618 (6.6432, -43.2495) -> (8.7265, -43.2495)
  line L619 (8.7265, -43.2495) -> (8.7265, -40.3329)
  line L620 (8.7265, -40.3329) -> (9.5598, -40.3329)
  line L621 (9.5598, -40.3329) -> (9.5598, -44.0829)
  line L622 (9.5598, -44.0829) -> (2.8932, -44.0829)
  line L623 (2.8932, -44.0829) -> (2.8932, -40.3329)
  line L624 (2.8932, -32.8329) -> (3.7265, -32.8329)
  line L625 (3.7265, -32.8329) -> (3.7265, -36.5829)
  line L626 (3.7265, -36.5829) -> (4.1432, -36.5829)
  line L627 (4.1432, -36.5829) -> (4.1432, -36.9995)
  line L628 (4.1432, -36.9995) -> (4.9765, -36.9995)
  line L629 (4.9765, -36.9995) -> (4.9765, -36.5829)
  line L630 (4.9765, -36.5829) -> (5.3932, -36.5829)
  line L631 (5.3932, -36.5829) -> (5.3932, -36.1662)
  line L632 (5.3932, -36.1662) -> (5.8098, -36.1662)
  line L633 (5.8098, -36.1662) -> (5.8098, -34.0829)
  line L634 (5.8098, -34.0829) -> (6.6432, -34.0829)
  line L635 (6.6432, -34.0829) -> (6.6432, -33.6662)
  line L636 (6.6432, -33.6662) -> (7.0598, -33.6662)
  line L637 (7.0598, -33.6662) -> (7.0598, -33.2495)
  line L638 (7.0598, -33.2495) -> (7.4765, -33.2495)
  line L639 (7.4765, -33.2495) -> (7.4765, -32.8329)
  line L640 (7.4765, -32.8329) -> (8.3098, -32.8329)
  line L641 (8.3098, -32.8329) -> (8.3098, -33.2495)
  line L642 (8.3098, -33.2495) -> (8.7265, -33.2495)
  line L643 (8.7265, -33.2495) -> (8.7265, -33.6662)
  line L644 (8.7265, -33.6662) -> (9.1432, -33.6662)
  line L645 (9.1432, -33.6662) -> (9.1432, -34.0829)
  line L646 (9.1432, -34.0829) -> (9.5598, -34.0829)
  line L647 (9.5598, -34.0829) -> (9.5598, -37.8329)
  line L648 (9.5598, -37.8329) -> (8.7265, -37.8329)
  line L649 (8.7265, -37.8329) -> (8.7265, -34.0829)
  line L650 (8.7265, -34.0829) -> (8.3098, -34.0829)
  line L651 (8.3098, -34.0829) -> (8.3098, -33.6662)
  line L652 (8.3098, -33.6662) -> (7.4765, -33.6662)
  line L653 (7.4765, -33.6662) -> (7.4765, -34.0829)
  line L654 (7.4765, -34.0829) -> (7.0598, -34.0829)
  line L655 (7.0598, -34.0829) -> (7.0598, -34.4995)
  line L656 (7.0598, -34.4995) -> (6.6432, -34.4995)
  line L657 (6.6432, -34.4995) -> (6.6432, -36.1662)
  line L658 (6.6432, -36.1662) -> (6.2265, -36.1662)
  line L659 (6.2265, -36.1662) -> (6.2265, -36.5829)
  line L660 (6.2265, -36.5829) -> (5.8098, -36.5829)
  line L661 (5.8098, -36.5829) -> (5.8098, -36.9995)
  line L662 (5.8098, -36.9995) -> (5.3932, -36.9995)
  line L663 (5.3932, -36.9995) -> (5.3932, -37.4162)
  line L664 (5.3932, -37.4162) -> (4.9765, -37.4162)
  line L665 (4.9765, -37.4162) -> (4.9765, -37.8329)
  line L666 (4.9765, -37.8329) -> (4.1432, -37.8329)
  line L667 (4.1432, -37.8329) -> (4.1432, -37.4162)
  line L668 (4.1432, -37.4162) -> (3.7265, -37.4162)
  line L669 (3.7265, -37.4162) -> (3.7265, -36.9995)
  line L670 (3.7265, -36.9995) -> (3.3098, -36.9995)
  line L671 (3.3098, -36.9995) -> (3.3098, -36.5829)
  line L672 (3.3098, -36.5829) -> (2.8932, -36.5829)
  line L673 (2.8932, -36.5829) -> (2.8932, -32.8329)
  line L674 (3.7265, -57.4162) -> (4.1432, -57.4162)
  line L675 (4.1432, -57.4162) -> (4.1432, -57.8329)
  line L676 (4.1432, -57.8329) -> (4.5598, -57.8329)
  line L677 (4.5598, -57.8329) -> (4.5598, -58.2495)
  line L678 (4.5598, -58.2495) -> (7.4765, -58.2495)
  line L679 (7.4765, -58.2495) -> (7.4765, -56.1662)
  line L680 (7.4765, -56.1662) -> (4.5598, -56.1662)
  line L681 (4.5598, -56.1662) -> (4.5598, -56.5829)
  line L682 (4.5598, -56.5829) -> (4.1432, -56.5829)
  line L683 (4.1432, -56.5829) -> (4.1432, -56.9995)
  line L684 (4.1432, -56.9995) -> (3.7265, -56.9995)
  line L685 (3.7265, -56.9995) -> (3.7265, -57.4162)
  line L686 (4.5598, -56.9995) -> (4.9765, -56.9995)
  line L687 (4.9765, -56.9995) -> (4.9765, -56.5829)
  line L688 (4.9765, -56.5829) -> (7.0598, -56.5829)
  line L689 (7.0598, -56.5829) -> (7.0598, -57.8329)
  line L690 (7.0598, -57.8329) -> (4.9765, -57.8329)
  line L691 (4.9765, -57.8329) -> (4.9765, -57.4162)
  line L692 (4.9765, -57.4162) -> (4.5598, -57.4162)
  line L693 (4.5598, -57.4162) -> (4.5598, -56.9995)
extrude "Extrude6" add sketch "Sketch2" along normal blind 1 separate body contours A1 L11 L12 L13 L14 L15 L16 L17 L18 L19 L120 L121 L122 L123 L124 L125 L126 L127 L135 L136 L137 | A1 L0 L1 L2 L3 L4 L5 L6 L7 L8 L9 L10 L11 L19 L128 L129 L130 L131 L132 L133 L134 L135 | A1 L120 L121 L122 L123 L124 L125 L126 L127 L129 L130 L131 L132 L133 L134 L135 L136 L137 | A1 L134 L135 | A1 L133 L134 | A1 L132 L133 | A1 L324 L325 L326 L327 L328 L329 L330 L331 L332 L333 L513 L514 L515 L516 L517 L518 L519 L520 L521 L522 | A1 L316 L317 L318 L319 L320 L321 L322 L323 L324 L333 L334 L335 L336 L337 L338 L339 L340 L341 L342 L343 L344 L345 L346 L347 L348 L349 L350 L351 L352 L353 L354 L355 L356 L357 L358 L359 L360 L361 L486 L487 L488 L489 L490 L491 L492 L493 L494 L495 L496 L497 L498 L499 L500 L501 L502 L503 L504 L505 L506 L507 L508 L509 L510 L511 L512 L513 L522 L523 L524 L525 L526 L527 L528 L529 L530 L531 | A1 L131 L132 | A1 L513 L514 | A1 L486 L487 L488 L489 L490 L491 L492 L493 L494 L495 L496 L497 L498 L499 L500 L501 L502 L503 L504 L505 L506 L507 L508 L509 L510 L511 L512 L513 L514 L515 L522 L523 L524 L525 L526 L527 L528 L529 L530 L531 | A1 L130 L131 | A1 L514 L515 | A1 L129 L130 | A1 L515 L516 L517 L518 L519 L520 L521 L522 | A1 L128 L129 | L20 L21 L22 L23 L24 L25 L26 L27 L28 L29 L30 L31 L32 L33 L34 L35 L36 L37 L38 L39 L40 L41 L42 L43 L44 L45 L46 L47 L48 L49 L50 L51 L52 L53 L54 L55 L56 L57 L58 L59 L60 L61 L62 L63 L64 L65 L66 L67 L68 L69 L70 L71 L72 L73 L74 L75 | L76 L77 L78 L79 L80 L81 L82 L83 L84 L85 L86 L87 L88 L89 L90 L91 L92 L93 L94 L95 L96 L97 L98 L99 | L100 L101 L102 L103 L104 L105 L106 L107 L108 L109 L110 L111 | L112 L113 L114 L115 L116 L117 L118 L119 | L138 L139 L140 L141 L142 L143 L144 L145 L146 L147 L148 L149 L150 L151 L152 L153 L154 L155 L156 L157 L158 L159 L160 L161 L162 L163 L164 L165 L166 L167 L168 L169 L170 L171 L172 L173 L174 L175 L176 L177 L178 L179 L180 L181 L182 L183 L184 L185 L186 L187 L188 L189 L190 L191 L192 L193 L194 L195 | L196 L197 L198 L199 L200 L201 L202 L203 L204 L205 L206 L207 L208 L209 L210 L211 L212 L213 L214 L215 L216 L217 L218 L219 L220 L221 L222 L223 | L224 L225 L226 L227 L228 L229 L230 L231 L232 L233 L234 L235 | L236 L237 L238 L239 L240 L241 L242 L243 | L244 L245 L246 L247 L248 L249 L250 L251 | L252 L253 L254 L255 L256 L257 L258 L259 | L260 L261 L262 L263 L264 L265 L266 L267 L268 L269 L270 L271 L272 L273 L274 L275 L276 L277 L278 L279 | L280 L281 L282 L283 L284 L285 L286 L287 | L288 L289 L290 L291 L292 L293 L294 L295 L296 L297 L298 L299 L300 L301 L302 L303 L304 L305 L306 L307 | L308 L309 L310 L311 L312 L313 L314 L315 | L362 L363 L364 L365 L366 L367 L368 L369 L370 L371 L372 L373 L374 L375 L376 L377 L378 L379 L380 L381 L382 L383 L384 L385 | L386 L387 L388 L389 L390 L391 L392 L393 L394 L395 L396 L397 L398 L399 L400 L401 L402 L403 L404 L405 L406 L407 L408 L409 L410 L411 L412 L413 L414 L415 L416 L417 L418 L419 L420 L421 L422 L423 L424 L425 L426 L427 L428 L429 | L430 L431 L432 L433 L434 L435 L436 L437 L438 L439 L440 L441 | L624 L625 L626 L627 L628 L629 L630 L631 L632 L633 L634 L635 L636 L637 L638 L639 L640 L641 L642 L643 L644 L645 L646 L647 L648 L649 L650 L651 L652 L653 L654 L655 L656 L657 L658 L659 L660 L661 L662 L663 L664 L665 L666 L667 L668 L669 L670 L671 L672 L673 | L442 L443 L444 L445 L446 L447 L448 L449 L450 L451 L452 L453 L454 L455 L456 L457 L458 L459 L460 L461 L462 L463 L464 L465 L466 L467 L468 L469 L470 L471 L472 L473 L474 L475 L476 L477 L478 L479 L480 L481 L482 L483 L484 L485 | L532 L533 L534 L535 L536 L537 L538 L539 L540 L541 L542 L543 L544 L545 L546 L547 L548 L549 L550 L551 L552 L553 L554 L555 | L556 L557 L558 L559 L560 L561 L562 L563 L564 L565 L566 L567 L568 L569 L570 L571 L572 L573 L574 L575 L576 L577 L578 L579 L580 L581 L582 L583 L584 L585 L586 L587 L588 L589 L590 L591 L592 L593 L594 L595 L596 L597 L598 L599 L600 L601 L602 L603 L604 L605 L606 L607 L608 L609 L610 L611 | L612 L613 L614 L615 L616 L617 L618 L619 L620 L621 L622 L623 | L674 L675 L676 L677 L678 L679 L680 L681 L682 L683 L684 L685 | L686 L687 L688 L689 L690 L691 L692 L693 makes body 2 at (-1.1346, -55.6107, 0.4) makes body 3 at (9.421, -35.4718, 0.4) makes body 4 at (6.3654, -53.1107, 0.4) makes body 5 at (5.9487, -43.944, 0.4) makes body 6 at (-4.329, -49.3607, 0.4) makes body 7 at (-3.2179, -42.4162, 0.4) makes body 8 at (5.5321, -57.4162, 0.4) makes body 9 at (-5.9957, -63.1107, 0.4) makes body 10 at (-1.829, -35.7495, 0.4) makes body 11 at (6.6432, -66.444, 0.4)
move_body "Move1" bodies 9 2 7 10 3 6 5 4 8 11 to x (1, 0, 0) y (0, 1, 0) z (0, 0, 1) at (0, 8, 4)
extrude "Extrude7" cut 10 faces at (-5.9957, -55.1107, 4.4) (-1.1346, -47.6107, 4.4) (-4.329, -41.3607, 4.4) (-3.2179, -34.4162, 4.4) (-1.829, -27.7495, 4.4) (6.6432, -58.444, 4.4) (5.5321, -49.4162, 4.4) (6.3654, -45.1107, 4.4) (5.9487, -35.944, 4.4) (9.421, -27.4718, 4.4) along direction (0, 0, -1) blind 4.4 on bodies 2 3 4 5 6 7 8 9 10 11 bodies 1
sketch "Sketch4" plane through (0, 0, 2) normal (0, 0, 1) x (1, 0, 0)
  line L0 (13.2739, -11.25) -> (-13.2739, -11.25)
  arc A0 (-13.2739, 11.25) -> (-13.2739, -11.25) centre (0, 0) ccw
  line L1 (-13.2739, 11.25) -> (13.2739, 11.25)
  arc A1 (13.2739, -11.25) -> (13.2739, 11.25) centre (0, 0) ccw
  circle A2 centre (0, 0) radius 18.4
  line L2 (-13.2739, -11.25) -> (-24, -11.25)
  line L3 (-24, -11.25) -> (26, -11.25)
  line L4 (13.2739, 11.25) -> (29, 11.25)
  line L5 (29, 11.25) -> (-22, 11.25)
  constraint coincident L0.end A0.end
  constraint parallel L0 L2
  constraint parallel L0 L3
  constraint coincident L1.end A1.end
  constraint parallel L1 L4
  constraint parallel L1 L5
extrude "Extrude8" cut sketch "Sketch4" against normal blind 2 contours A1 A2 L3 L4 L5 | A0 A2 L2 L3 L5 bodies 1
move_face "OffsetFaces1" offset -0.1 2 faces at (-4.8534, 11.25, 0.9333) (-4.8534, -11.25, 0.9333) on bodies 1
equation "d2 = 36.800 mm / 8"
equation "d3 = 36.800 mm / 8"
equation "d7 = ( 22.5 / 2 ) * 1 mm"
